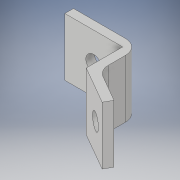
# Autodesk Inventor part: Acrylic_angle_bracket
Saved by Autodesk Inventor 2019.4 (Build 234330000, 330)
## iProperties
Created: 2020-02-04
Part Number: Acrylic_angle_bracket
Material: Generic
Document SubType Name: Modeling
Designer: Jorian Bruslind
Density: 1 g/cm^3
Appearance: Default
Author: Jorian Bruslind
Autodesk Inventor part; units mm, degrees
ref_plane "YZ Plane" through (0, 0, 0) normal (1, 0, 0) x (0, 1, 0)
ref_plane "XZ Plane" through (0, 0, 0) normal (0, 1, 0) x (-1, 0, 0)
ref_plane "XY Plane" through (0, 0, 0) normal (0, 0, 1) x (1, 0, 0)
sketch "Sketch4" plane through (0, 0, 0) normal (0, 1, 0) x (-1, 0, 0)
  line L0 (0, 0) -> (0, -12.6)
  line L1 (0, -12.6) -> (20, -12.6)
  line L2 (20, -12.6) -> (0, -12.6)
  line L3 (0, -12.6) -> (0, -15.6)
  line L4 (0, -15.6) -> (20, -15.6)
  line L5 (20, -15.6) -> (20, -12.6)
  line L6 (0, 0) -> (-12.9904, 7.5)
  line L7 (0, 0) -> (15, 0) construction
  line L8 (-12.9904, 7.5) -> (0, 0)
  line L9 (0, 0) -> (-1.5, -2.5981)
  line L10 (-1.5, -2.5981) -> (-14.4904, 4.9019)
  line L11 (-14.4904, 4.9019) -> (-12.9904, 7.5)
  line L12 (0, 0) -> (0, -15.6)
  line L13 (0, -15.6) -> (-3, -15.6)
  line L14 (-3, -15.6) -> (-3, 0)
  line L15 (-3, 0) -> (0, 0)
  dimension "d16" = 12.6
  dimension "d17" = 20
  dimension "d18" = 3
  dimension "d19" = 15
  dimension "d20" = 150
  dimension "d21" = 3
  dimension "d24" = 3
  constraints: 32 end point, 6 parallel, 4 perpendicular, 2 horizontal, 1 collinear, 1 equal length, 1 vertical
  measures "d16" distance of L0.start L0.end
  measures "d17" distance of L0.end L1.end
  measures "d18" distance of L3.end L0.end
  measures "d19" distance of L0.start L6.end
  measures "d20" angle of L7 L6
  measures "d21" distance of L0.start L9.end
  measures "d24" distance of L3.end L13.end
extrude "Extrusion5" add sketch "Sketch4" along normal blind 20
sketch "Sketch5" plane through (3, 0, -15.6) normal (0, 0, -1) x (-1, 0, 0)
  line L0 (3, 0) -> (23, 0) projected
  line L1 (13, 0) -> (13, 10)
  circle A0 centre (13, 10) radius 2.75
  dimension "d27" = 10
  dimension "d28" = 5.5
  constraints: 2 end point, 1 centre point, 1 coincident, 1 midpoint, 1 vertical
  measures "d27" distance of L1.start L1.end
  measures "d28" diameter of A0
extrude "Extrusion6" cut sketch "Sketch5" against normal blind 3
sketch "Sketch6" plane through (3, 0, -1.7321) normal (0.5, 0, -0.866) x (-0.866, 0, -0.5)
  line L0 (0, 0) -> (0, 20) projected
  line L1 (0, 10) -> (-7, 10)
  circle A0 centre (-7, 10) radius 2.75
  point P0 (1.7321, 0)
  dimension "d31" = 7
  dimension "d32" = 5.5
  constraints: 2 end point, 1 centre point, 1 coincident, 1 horizontal, 1 midpoint
  measures "d31" distance of L1.start L1.end
  measures "d32" diameter of A0
extrude "Extrusion7" cut sketch "Sketch6" against normal blind 3
fillet "Fillet1" radius 5 2 edges at (3, 10, -1.7321) (3, 10, -15.6)
body "Solid3"
